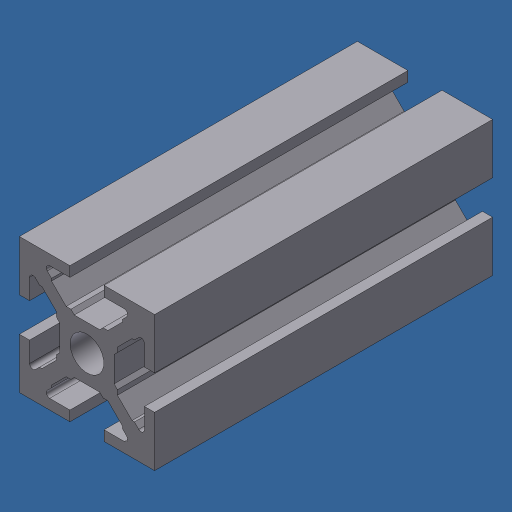
# Autodesk Inventor part: BAR, EXTRUDED ALUM, 40MMX40MM, MK, STD DUTY, 54_01 SERIES
Saved by Autodesk Inventor 2024.3 (Build 283343000, 343)
## iProperties
Category: _
Manager: _
RuleStatus: InUse
Shininess: 64.0
Angle Display Precision: 2
Document Length Units: 11269
Document Angle Units: 11279
Document Time Units: 11290
Document Mass Units: 11283
Document Length Units Precision: 3
Document Angle Units Precision: 2
Part Number: BAR, EXTRUDED ALUM, 40MMX40MM, MK, STD DUTY, 54_01 SERIES
Material: Aluminum, 6061-T6
Document SubType Name: Modeling
Created: 2019-07-31
Designer: -
Manufacturer: Standard
Standards Organization: Custom
Density: 2.71 g/cm^3
Description: BAR, MK EXTRUDED ALUM, 40MMX40MM
Checked By: 00
Engr Approved By: R
User Status: Work In Process
Mfg Approved By: -
Appearance: Aluminum (Flat)
Mass: 201.592 g
Surface Area: 378.284 cm^2
Volume: 74.3882 cm^3
BeforeDocSave0: Mass
BeforeDocSave1: PartFinishTrigger
Density: 0.0
Volumn: 0.0
Area: 0.0
PropertySet Name: Model Information
Control State: 0
Master: False
Checked Out: False
CN_MASS: 0.2
CN_SERVICEABLE: _
CL_runCount: 0
FIRST_DESCRIPTION: _
SECOND_DESCRIPTION: _
THIRD_DESCRIPTION: _
Author: -
Subject: _
Revision Number: A
Keywords: -
Autodesk Inventor part; units mm, degrees
ref_plane "YZ Plane" through (0, 0, 0) normal (1, 0, 0) x (0, 1, 0)
ref_plane "XZ Plane" through (0, 0, 0) normal (0, 1, 0) x (-1, 0, 0)
ref_plane "XY Plane" through (0, 0, 0) normal (0, 0, 1) x (1, 0, 0)
sketch "Sketch1" plane through (0, 0, 0) normal (0, 0, 1) x (1, 0, 0)
  arc A0 (0, 5) -> (-5, 0) centre (0, 0) ccw
  line L0 (-5.05, 20.0001) -> (-20, 20.0001)
  line L1 (-20, 20.0001) -> (-20, 5.0501)
  line L2 (-20, 5.0501) -> (-17, 5.0501)
  line L3 (-5.05, 20.0001) -> (-5.05, 17.0001)
  line L4 (0, 8) -> (-3.7572, 8)
  line L5 (-8, 3.7574) -> (-8, 0)
  arc A1 (-15.2929, 11.7574) -> (-17, 11.0503) centre (-16, 11.0503) ccw
  arc A2 (-11.0502, 17.0001) -> (-11.7573, 15.2929) centre (-11.0502, 16.0001) ccw
  line L6 (-17, 5.0501) -> (-17, 11.0503)
  line L7 (-5.05, 17.0001) -> (-11.0502, 17.0001)
  line L8 (-11.7573, 15.2929) -> (-5.4644, 9)
  line L9 (-15.2929, 11.7574) -> (-9, 5.4645)
  line L10 (0, 0) -> (-41.3511, 0) construction
  arc A3 (-5, 0) -> (0, -5) centre (0, 0) ccw
  line L11 (-5.05, -20.0001) -> (-20, -20.0001)
  line L12 (-20, -20.0001) -> (-20, -5.0501)
  line L13 (-20, -5.0501) -> (-17, -5.0501)
  line L14 (-5.05, -20.0001) -> (-5.05, -17.0001)
  line L15 (0, -8) -> (-3.7572, -8)
  line L16 (-8, -3.7574) -> (-8, 0)
  arc A4 (-17, -11.0503) -> (-15.2929, -11.7574) centre (-16, -11.0503) ccw
  arc A5 (-11.7573, -15.2929) -> (-11.0502, -17.0001) centre (-11.0502, -16.0001) ccw
  line L17 (-17, -5.0501) -> (-17, -11.0503)
  line L18 (-5.05, -17.0001) -> (-11.0502, -17.0001)
  line L19 (-11.7573, -15.2929) -> (-5.4644, -9)
  line L20 (-15.2929, -11.7574) -> (-9, -5.4645)
  line L21 (0, 26.9899) -> (0, -26.9183) construction
  arc A6 (0, -5) -> (5, 0) centre (0, 0) ccw
  line L22 (8, -3.7574) -> (8, 0)
  line L23 (15.2929, -11.7574) -> (9, -5.4645)
  line L24 (11.7573, -15.2929) -> (5.4644, -9)
  line L25 (0, -8) -> (3.7572, -8)
  line L26 (5.05, -17.0001) -> (11.0502, -17.0001)
  arc A7 (11.0502, -17.0001) -> (11.7573, -15.2929) centre (11.0502, -16.0001) ccw
  line L27 (5.05, -20.0001) -> (5.05, -17.0001)
  line L28 (5.05, -20.0001) -> (20, -20.0001)
  line L29 (20, -20.0001) -> (20, -5.0501)
  line L30 (20, -5.0501) -> (17, -5.0501)
  line L31 (17, -5.0501) -> (17, -11.0503)
  arc A8 (15.2929, -11.7574) -> (17, -11.0503) centre (16, -11.0503) ccw
  arc A9 (5, 0) -> (0, 5) centre (0, 0) ccw
  line L32 (20, 5.0501) -> (20, 20.0001)
  line L33 (5.05, 20.0001) -> (20, 20.0001)
  line L34 (5.05, 20.0001) -> (5.05, 17.0001)
  line L35 (20, 5.0501) -> (17, 5.0501)
  line L36 (5.4644, 9) -> (11.7573, 15.2929)
  line L37 (9, 5.4645) -> (15.2929, 11.7574)
  line L38 (5.05, 17.0001) -> (11.0502, 17.0001)
  line L39 (17, 5.0501) -> (17, 11.0503)
  arc A10 (11.7573, 15.2929) -> (11.0502, 17.0001) centre (11.0502, 16.0001) ccw
  arc A11 (17, 11.0503) -> (15.2929, 11.7574) centre (16, 11.0503) ccw
  line L40 (-3.7572, 8) -> (-4.7572, 9)
  line L41 (-8, 3.7574) -> (-9, 4.7574)
  line L42 (-9, 4.7574) -> (-9, 5.4645)
  line L43 (-4.7572, 9) -> (-5.4644, 9)
  line L44 (-3.7572, -8) -> (-4.7572, -9)
  line L45 (-8, -3.7574) -> (-9, -4.7574)
  line L46 (-9, -4.7574) -> (-9, -5.4645)
  line L47 (-4.7572, -9) -> (-5.4644, -9)
  line L48 (3.7572, 8) -> (4.7572, 9)
  line L49 (8, 3.7574) -> (9, 4.7574)
  line L50 (9, 4.7574) -> (9, 5.4645)
  line L51 (4.7572, 9) -> (5.4644, 9)
  line L52 (8, -3.7574) -> (9, -4.7574)
  line L53 (9, -4.7574) -> (9, -5.4645)
  line L54 (4.7572, -9) -> (5.4644, -9)
  line L55 (3.7572, -8) -> (4.7572, -9)
  line L56 (0, 8) -> (3.7572, 8)
  line L57 (8, 3.7574) -> (8, 0)
  point P0 (-4.4644, 8)
  point P1 (-8, 4.4645)
  dimension "d0" = 10
  dimension "d3" = 14.95
  dimension "d4" = 14.95
  dimension "d5" = 3
  dimension "d7" = 2
  dimension "d8" = 4
  dimension "d9" = 4
  dimension "d10" = 8.9498
  dimension "d11" = 8.9498
  dimension "d12" = 45
  dimension "d16" = 8
  dimension "d18" = 2.5
  dimension "d19" = 20
  dimension "d21" = 1
  dimension "d24" = 0.5
  dimension "d25" = 0.5
  dimension "d26" = 1
  dimension "d34" = 8
  constraints: 116 end point, 44 symmetric about line, 24 point on circle, 13 perpendicular, 12 centre point, 8 parallel, 8 tangent, 5 horizontal alignment, 4 vertical alignment, 3 equal length, 2 coincident, 2 equal radius, 1 horizontal, 38 other
  measures "d0" diameter of A0
  measures "d3" distance between parallel lines of L1 L3
  measures "d4" distance between parallel lines of L0 L2
  measures "d5" distance of L1.end L2.end
  measures "d7" diameter of A1
  measures "d8" distance from line of L1 A1.centre
  measures "d9" distance from line of L0 A2.centre
  measures "d10" distance from line of L0 A1.centre
  measures "d11" distance from line of L1 A2.centre
  measures "d12" angle of L7 L8
  measures "d16" distance from line of A0.centre L5
  measures "d18" distance from line of A0.centre L9
  measures "d19" distance from line of A0.centre L1
  measures "d21" radius of A10
  measures "d24" distance between parallel lines of L8 L40
  measures "d25" distance between parallel lines of L41 L9
  measures "d26" distance from line of L4 L40.end
  measures "d34" distance from line of A0.centre L56
extrude "MK, 40X40" add sketch "Sketch1" along normal blind 100
sketch "Sketch2" plane through (0, 0, 100) normal (0, 0, 1) x (1, 0, 0)
  circle A0 centre (0, 0) radius 5 projected
  line L0 (-9, 5.4645) -> (-15.2929, 11.7574) projected
  line L1 (-11.7573, 15.2929) -> (-5.4644, 9) projected
  line L2 (-13.3283, 10.5) -> (-9, 6.1717)
  line L3 (-6.1715, 9) -> (-10.5, 13.3285)
  line L4 (-5.4644, 9) -> (-6.1715, 9)
  line L5 (-5.4644, 9) -> (-4.7572, 9) projected
  line L6 (-9, 5.4645) -> (-9, 6.1717)
  line L7 (-10.5, 14.0356) -> (-10.5, 13.3285)
  line L8 (-13.3283, 10.5) -> (-14.0355, 10.5)
  line L9 (0, 0) -> (-37.9325, 0) construction
  line L10 (0, 26.9937) -> (0, -28.1119) construction
  line L11 (-13.3283, -10.5) -> (-9, -6.1717)
  line L12 (-6.1715, -9) -> (-10.5, -13.3285)
  line L13 (-5.4644, -9) -> (-6.1715, -9)
  line L14 (-9, -5.4645) -> (-9, -6.1717)
  line L15 (-10.5, -14.0356) -> (-10.5, -13.3285)
  line L16 (-13.3283, -10.5) -> (-14.0355, -10.5)
  line L17 (13.3283, 10.5) -> (9, 6.1717)
  line L18 (6.1715, 9) -> (10.5, 13.3285)
  line L19 (5.4644, 9) -> (6.1715, 9)
  line L20 (9, 5.4645) -> (9, 6.1717)
  line L21 (10.5, 14.0356) -> (10.5, 13.3285)
  line L22 (13.3283, 10.5) -> (14.0355, 10.5)
  line L23 (13.3283, -10.5) -> (14.0355, -10.5)
  line L24 (13.3283, -10.5) -> (9, -6.1717)
  line L25 (9, -5.4645) -> (9, -6.1717)
  line L26 (5.4644, -9) -> (6.1715, -9)
  line L27 (6.1715, -9) -> (10.5, -13.3285)
  line L28 (10.5, -14.0356) -> (10.5, -13.3285)
  line L29 (-14.0355, -10.5) -> (-9, -5.4645)
  line L30 (-15.2929, -11.7574) -> (-9, -5.4645) projected
  line L31 (-5.4644, -9) -> (-10.5, -14.0356)
  line L32 (-5.4644, -9) -> (-11.7573, -15.2929) projected
  line L33 (10.5, -14.0356) -> (5.4644, -9)
  line L34 (14.0355, -10.5) -> (9, -5.4645)
  line L35 (9, 5.4645) -> (14.0355, 10.5)
  line L36 (10.5, 14.0356) -> (5.4644, 9)
  dimension "d28" = 4
  dimension "d29" = 0.5
  dimension "d30" = 10.5
  dimension "d31" = 10.5
  constraints: 64 end point, 18 symmetric about line, 5 parallel, 3 collinear, 3 perpendicular, 2 point on line, 18 other
  measures "d28" distance between parallel lines of L2 L3
  measures "d29" distance between parallel lines of L1 L3
  measures "d30" distance from line of L9.start L7
  measures "d31" distance from line of L8 L9.start
extrude "Extrusion2" cut sketch "Sketch2" against normal through all contours L0 L8 L2 L6 | L1 L4 L3 L7 | L16 L29 L14 L11 | L13 L31 L15 L12 | L22 L35 L20 L17 | L19 L36 L21 L18 | L24 L25 L34 L23 | L26 L27 L28 L33
equation "\"d4\" = d3"
